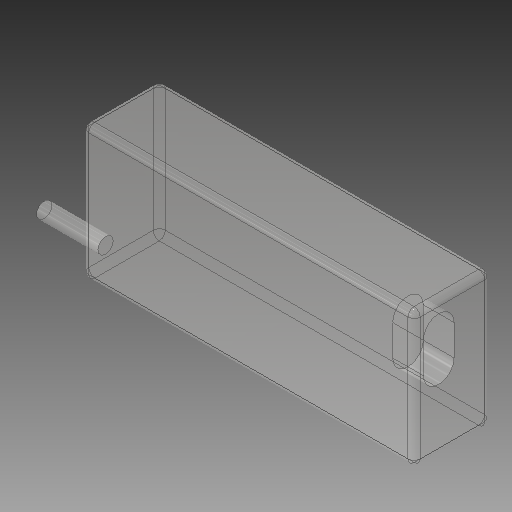
# Autodesk Inventor part: Transformer
Saved by Autodesk Inventor 2019 (Build 230136000, 136)
## iProperties
Created: 2018-12-20
Part Number: Transformer
Material: PET Plastic
Document SubType Name: Modeling
Designer: assman
Density: 1.541 g/cm^3
Appearance: Polycarbonate - Clear
Author: assman
Autodesk Inventor part; units mm, degrees
ref_plane "YZ Plane" through (0, 0, 0) normal (1, 0, 0) x (0, 1, 0)
ref_plane "XZ Plane" through (0, 0, 0) normal (0, 1, 0) x (-1, 0, 0)
ref_plane "XY Plane" through (0, 0, 0) normal (0, 0, 1) x (1, 0, 0)
sketch "Sketch1" plane through (0, 0, 0) normal (0, 0, 1) x (1, 0, 0)
  line L0 (54, 22) -> (-54, 22)
  line L1 (-54, 22) -> (-54, -22)
  line L2 (-54, -22) -> (54, -22)
  line L3 (54, -22) -> (54, 22)
  line L4 (-54, 0) -> (54, 0) construction
  line L5 (0, 22) -> (0, -22) construction
  point P0 (0, 0)
  point P1 (0, 0)
  dimension "d0" = 108
  dimension "d1" = 44
  constraints: 12 end point, 5 midpoint, 2 parallel, 1 coincident, 1 horizontal, 1 perpendicular
  measures "d0" distance of L2.end L1.end
  measures "d1" distance of L1.end L0.end
extrude "Extrusion1" add sketch "Sketch1" along normal blind 25
fillet "Fillet1" radius 2 9 edges at (0, 22, 25) (0, -22, 25) (0, -22, 0) (0, 22, 0) (54, 0, 0) (54, 22, 12.5) (54, -22, 12.5) (-54, 0, 25) (-54, 0, 0)
sketch "Sketch2" plane through (54, -20, 2) normal (1, 0, 0) x (0, 0, -1)
  line L0 (0, 0) -> (-23, 0) construction
  line L1 (0, 40) -> (0, 0) construction
  line L2 (-23, 40) -> (0, 40) construction
  line L3 (-23, 0) -> (-23, 40) construction
  line L4 (-20, 18) -> (-10, 18)
  line L5 (-10, 18) -> (-10, 38)
  line L6 (-10, 38) -> (-20, 38)
  line L7 (-20, 38) -> (-20, 18)
  point P0 (2, 20)
  dimension "d5" = 10
  dimension "d6" = 20
  dimension "d7" = 3
  dimension "d8" = 18
  constraints: 8 end point, 2 parallel, 1 horizontal, 1 perpendicular
  measures "d5" distance of L6.end L5.end
  measures "d6" distance of L5.end L4.end
  measures "d7" distance between parallel lines of L7 L3
  measures "d8" distance between parallel lines of L0 L4
extrude "Extrusion2" cut sketch "Sketch2" against normal blind 10
sketch "Sketch3" plane through (-54, -22, 23) normal (-1, 0, 0) x (0, 0, 1)
  line L0 (0, 44) -> (0, 0) construction
  line L1 (-21, 0) -> (0, 0) construction
  circle A0 centre (-5.5, 5.5) radius 2.5
  point P0 (-23, 22)
  dimension "d11" = 5
  dimension "d13" = 3
  dimension "d14" = 3
  constraints: 1 centre point
  measures "d11" diameter of A0
  measures "d13" distance edge to line of A0 L0
  measures "d14" distance edge to line of A0 L1
extrude "Extrusion3" add sketch "Sketch3" along normal blind 20
fillet "Fillet2" radius 2 3 edges at (53.4142, 21.4142, 24.4142) (53.4142, -21.4142, 24.4142) (54, 0, 25)
fillet "Fillet3" radius 5 1 edges at (49, -2, 22)
fillet "Fillet4" radius 5 3 edges at (49, 18, 22) (49, 18, 12) (49, -2, 12)
fillet "Fillet5" radius 2 6 edges at (-53.4142, 21.4142, 24.4142) (-53.4142, 21.4142, 0.5858) (-54, 22, 12.5) (-53.4142, -21.4142, 24.4142) (-53.4142, -21.4142, 0.5858) (-54, -22, 12.5)
body "Solid1"
